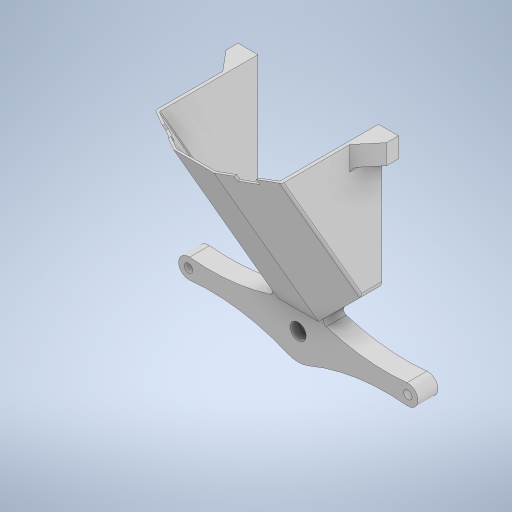
# Autodesk Inventor part: Brida_Rodamiento_Inferior
Saved by Autodesk Inventor 2024 (Build 280153000, 153)
## iProperties
Created: 2024-07-16
Part Number: Brida_Rodamiento_Inferior
Material: Genérico
Document SubType Name: Modeling
Designer: sergi
Density: 1 g/cm^3
Appearance: Valor por defecto
Author: sergi
Autodesk Inventor part; units mm, degrees
sketch "Boceto1" plane through (0, 0, 0) normal (0, 0, 1) x (1, 0, 0)
  circle A0 centre (0, 0) radius 8.25
  arc A1 (-36.764317, -25.949663) -> (36.764317, -25.949663) centre (0, 0) ccw
  arc A2 (-35.575624, -20.539596) -> (-36.764317, -25.949663) centre (-33.700624, -23.787191) ccw
  line L0 (-35.575624, -20.539596) -> (-15.909903, -9.185587)
  arc A3 (-11.227922, -9.946545) -> (-15.909903, -9.185587) centre (-14.034903, -12.433182) ccw
  arc A4 (-11.227922, -9.946545) -> (11.227922, -9.946545) centre (0, 0) ccw
  arc A5 (15.909903, -9.185587) -> (11.227922, -9.946545) centre (14.034903, -12.433182) ccw
  line L1 (15.909903, -9.185587) -> (35.575624, -20.539596)
  arc A6 (36.764317, -25.949663) -> (35.575624, -20.539596) centre (33.700624, -23.787191) ccw
  line L2 (98, -98) -> (98, 98)
  line L3 (98, 98) -> (-98, 98)
  line L4 (-98, 98) -> (-98, -98)
  line L5 (-98, -98) -> (98, -98)
  circle A7 centre (0, 0) radius 4
  line L6 (21.465456, -12.393087) -> (15.909903, -9.185587)
  arc A8 (15.909903, -9.185587) -> (11.227922, -9.946545) centre (14.034903, -12.433182) ccw
  arc A9 (-11.227922, -9.946545) -> (11.227922, -9.946545) centre (0, 0) ccw
  arc A10 (-11.227922, -9.946545) -> (-15.909903, -9.185587) centre (-14.034903, -12.433182) ccw
  line L7 (-15.909903, -9.185587) -> (-21.465456, -12.393087)
  line L8 (0, 0) -> (-55, 0) construction
  line L9 (0, 0) -> (55, 0) construction
  circle A11 centre (-55, 0) radius 2.1
  circle A12 centre (0, 0) radius 4
  circle A13 centre (-55, 0) radius 5
  circle A14 centre (0, 0) radius 13.4
  circle A15 centre (44.177818, -104.440798) radius 100
  circle A16 centre (-44.177818, -104.440798) radius 100
  arc A17 (0, 14.728367) -> (-5.220307, 12.341329) centre (-44.177818, 104.440798) ccw
  arc A18 (5.220307, 12.341329) -> (0, 14.728367) centre (44.177818, 104.440798) ccw
  line L10 (0, 0) -> (55, 0) construction
  circle A19 centre (55, 0) radius 5
  circle A20 centre (55, 0) radius 2.1
  line L11 (21.465456, -12.393087) -> (21.465456, 21.465456)
  line L12 (-21.465456, 21.465456) -> (-21.465456, -12.393087)
  line L13 (21.465456, 21.465456) -> (-21.465456, 21.465456)
  line L14 (-5.220307, 12.341329) -> (5.220307, 12.341329)
  line L15 (-11.631275, 9.885405) -> (11.631275, 9.885405)
  point P0 (0, 0)
  point P1 (21.81811, -12.596691)
  point P2 (-21.81811, -12.596691)
  point P3 (-11.631275, -9.46777)
  point P4 (-6.195652, 13.66067)
  point P5 (-54.484658, 4.973371)
  point P6 (-54.484658, -4.973371)
  point P7 (-14.969491, -8.801509)
  point P8 (14.969491, -8.801509)
  point P9 (6.195652, 13.66067)
  point P10 (27.999715, -35.228056)
  point P11 (-27.999715, -35.228056)
  point P12 (-11.125454, -10.061027)
  point P13 (11.125454, -10.061027)
  point P14 (11.227922, -9.946545)
  point P15 (11.227922, -9.946545)
  point P16 (54.484658, -4.973371)
  point P17 (54.484658, 4.973371)
  point P18 (25.599802, 0)
  point P19 (43.945653, 0)
  point P20 (-43.945653, 0)
  point P21 (-25.599802, 0)
  point P22 (-5.220307, -12.341329)
  point P23 (5.220307, -12.341329)
  point P24 (0, 192.73038)
  point P25 (0, 194.15323)
  point P26 (0, -194.15323)
  point P27 (0, -14.728367)
  point P28 (0.528736, -14.990678)
  point P29 (-0.528736, -14.990678)
  dimension "d3" = 180
  dimension "d4" = 4.2
  dimension "d16" = 10
  dimension "d18" = 55
  dimension "d19" = 26.8
  dimension "empalme" = 200
  dimension "d22" = 200
  dimension "d23" = 200
  dimension "d24" = 200
  dimension "d27" = 55
  dimension "d28" = 10
  dimension "d29" = 4.2
  constraints: 10 centre point, 10 end point, 8 point on circle, 8 tangent, 6 coincident, 3 horizontal, 1 collinear, 1 concentric, 1 point on line
  measures "d3" angle of L8 L9
  measures "d4" diameter of A11
  measures "d16" diameter of A13
  measures "d18" distance of L8.start L8.end
  measures "d19" diameter of A14
  measures "empalme" diameter of A15
  measures "d22" diameter of A16
  measures "d23" diameter of A17
  measures "d24" diameter of A18
  measures "d27" distance of L10.start L10.end
  measures "d28" diameter of A19
  measures "d29" diameter of A20
extrude "Extrusión1" add sketch "Boceto1" along normal blind 10 contours A0 | A15 L11 A18 A19 | A16 A3 A4 | A4 A3 A16 L12 A17 L15 A14 | A16 A13 A17 L12 | A15 A14 L15 A18 L11 A5 A4 | A4 A5 A15 | A14 L15 | A13 | A19
sketch "Boceto2" plane through (0, 0, 0) normal (0, 0, -1) x (-1, 0, 0)
  circle A0 centre (0, 0) radius 8.25 projected
  point P0 (0, 0)
extrude "Extrusión2" cut sketch "Boceto2" against normal blind 5
sketch "Boceto3" plane through (0, 0, 5) normal (0, 0, -1) x (-1, 0, 0)
  circle A0 centre (0, 0) radius 5.25 projected
  point P0 (0, 0)
extrude "Extrusión3" cut sketch "Boceto3" against normal blind 0.5
ref_plane "Plano de trabajo1" through (0, 0, 0) normal (0, 0, 1) x (1, 0, 0)
sketch "Boceto4" plane through (0, 0, 0) normal (0, 0, 1) x (1, 0, 0)
  line L0 (-31.810181, 100) -> (-31.810181, 32.452822)
  arc A0 (-31.810181, 32.452822) -> (-30.755766, 29.907238) centre (-28.210181, 32.452822) ccw
  line L1 (-30.755766, 29.907238) -> (-10.733933, 9.885405)
  line L2 (10.733933, 9.885405) -> (10.733933, 100)
  line L3 (30.755766, 29.907238) -> (30.755766, 100)
  line L4 (30.755766, 29.907238) -> (10.733933, 9.885405)
  line L5 (30.755766, 29.907238) -> (30.755766, 100)
  line L6 (-30.210181, 32.452822) -> (-30.210181, 100)
  arc A1 (-30.210181, 32.452822) -> (-29.624395, 31.038609) centre (-28.210181, 32.452822) ccw
  line L7 (-9.875898, 11.290112) -> (-29.624395, 31.038609)
  line L8 (9.875898, 11.290112) -> (-9.875898, 11.290112)
  line L9 (11.631275, 9.885405) -> (-11.631275, 9.885405)
  line L10 (29.624395, 31.038609) -> (9.875898, 11.290112)
  arc A2 (29.624395, 31.038609) -> (30.210181, 32.452822) centre (28.210181, 32.452822) ccw
  line L11 (30.210181, 100) -> (30.210181, 32.452822)
  line L12 (100, 100) -> (-100, 100)
  line L13 (31.810181, 32.452822) -> (31.810181, 100)
  arc A3 (30.755766, 29.907238) -> (31.810181, 32.452822) centre (28.210181, 32.452822) ccw
  line L14 (11.631275, 9.885405) -> (11.631275, 10.782746)
  line L15 (-11.631275, 9.885405) -> (-11.631275, 10.782746)
  point P0 (0, 0)
  point P1 (10.733933, 12.148146)
  constraints: 4 end point, 2 point on line, 1 parallel, 1 vertical
extrude "Extrusión4" add sketch "Boceto4" along normal up to surface (10 mm away) contours L12 L6 A1 L7 L8 L10 L2 L9 L1 A0 L0 | L1 L9 L15 | L10 A2 L11 L12 L3 L4 L2 | L4 L14 L9 | L12 L13 A3 L3
fillet "Empalme2" radius 2 4 edges at (-11.6313, 9.8854, 5) (-11.6313, 10.7827, 5) (11.6313, 9.8854, 5) (11.6313, 10.7827, 5)
sketch "Boceto5" plane through (0, 0, 10) normal (0, 0, 1) x (1, 0, 0)
  line L0 (-10.13864, 9.290112) -> (-30.755766, 29.907238)
  arc A0 (-31.810181, 32.452822) -> (-30.755766, 29.907238) centre (-28.210181, 32.452822) ccw
  arc A1 (-30.210181, 32.452822) -> (-29.624395, 31.038609) centre (-28.210181, 32.452822) ccw
  line L1 (-29.624395, 31.038609) -> (-9.875898, 11.290112)
  line L2 (-9.875898, 11.290112) -> (9.875898, 11.290112)
  line L3 (9.875898, 11.290112) -> (29.624395, 31.038609)
  line L4 (30.755766, 29.907238) -> (10.13864, 9.290112)
  arc A2 (30.755766, 29.907238) -> (31.810181, 32.452822) centre (28.210181, 32.452822) ccw
  line L5 (-103, 100) -> (100, 100)
  arc A3 (-54.484658, 4.973371) -> (-11.631275, 9.885405) centre (-44.177818, 104.440798) ccw
  arc A4 (-54.484658, 4.973371) -> (-11.631275, 9.885405) centre (-44.177818, 104.440798) ccw
  arc A5 (13.415067, 9.290112) -> (54.484658, 4.973371) centre (44.177818, 104.440798) ccw
  line L6 (11.631275, 10.782746) -> (11.631275, 9.885405)
  line L7 (-11.631275, 9.885405) -> (-11.631275, 10.782746)
  arc A6 (-54.484658, 4.973371) -> (-14.064455, 9.082603) centre (-44.177818, 104.440798) ccw
  arc A7 (-54.484658, 4.973371) -> (-54.484658, -4.973371) centre (-55, 0) ccw
  arc A8 (-5.220307, -12.341329) -> (-54.484658, -4.973371) centre (-44.177818, -104.440798) ccw
  arc A9 (-5.220307, -12.341329) -> (5.220307, -12.341329) centre (0, 0) ccw
  arc A10 (54.484658, -4.973371) -> (5.220307, -12.341329) centre (44.177818, -104.440798) ccw
  arc A11 (54.484658, -4.973371) -> (54.484658, 4.973371) centre (55, 0) ccw
  arc A12 (14.064455, 9.082603) -> (54.484658, 4.973371) centre (44.177818, 104.440798) ccw
  circle A13 centre (0, 0) radius 4
  line L8 (-14.064455, 9.082603) -> (-14.015792, 9.098659)
  line L9 (0, 11.290112) -> (0, 9.290112)
  line L10 (0, 9.290112) -> (-13.415067, 9.290112)
  line L11 (0, 9.290112) -> (13.415067, 9.290112)
  line L12 (30.755766, 29.907238) -> (13.252509, 12.403981)
  arc A14 (30.755766, 29.907238) -> (31.810181, 32.452822) centre (28.210181, 32.452822) ccw
  line L13 (31.810181, 100) -> (31.810181, 32.452822)
  line L14 (30.210181, 100) -> (31.810181, 100)
  line L15 (30.210181, 32.452822) -> (30.210181, 100)
  arc A15 (29.624395, 31.038609) -> (30.210181, 32.452822) centre (28.210181, 32.452822) ccw
  line L16 (9.875898, 11.290112) -> (29.624395, 31.038609)
  line L17 (-9.875898, 11.290112) -> (9.875898, 11.290112)
  line L18 (-29.624395, 31.038609) -> (-9.875898, 11.290112)
  arc A16 (-30.210181, 32.452822) -> (-29.624395, 31.038609) centre (-28.210181, 32.452822) ccw
  line L19 (-30.210181, 100) -> (-30.210181, 32.452822)
  line L20 (-31.810181, 100) -> (-30.210181, 100)
  line L21 (-31.810181, 32.452822) -> (-31.810181, 100)
  arc A17 (-31.810181, 32.452822) -> (-30.755766, 29.907238) centre (-28.210181, 32.452822) ccw
  line L22 (-13.252509, 12.403981) -> (-30.755766, 29.907238)
  arc A18 (-14.064455, 9.082603) -> (-13.252509, 12.403981) centre (-14.666723, 10.989767) ccw
  arc A19 (13.252509, 12.403981) -> (14.064455, 9.082603) centre (14.666723, 10.989767) ccw
  point P0 (0, 0)
  point P1 (-31.810181, 100)
  point P2 (-30.210181, 100)
  point P3 (30.210181, 100)
  point P4 (31.810181, 100)
  point P5 (-31.810181, 32.452822)
  dimension "d59" = 2
  constraints: 12 end point, 4 point on circle, 2 point on line, 1 centre point, 1 horizontal, 1 perpendicular
  measures "d59" distance of L9.start L9.end
ref_plane "Plano de trabajo2" through (0, 32.452822, 0) normal (-1, 0, 0) x (0, 0, 1)
sketch "Boceto6" plane through (0, 32.452822, 0) normal (-1, 0, 0) x (0, 0, 1)
  line L0 (10, -23.16271) -> (81, 99.812897)
  point P0 (10, 67.547178)
  constraints: 2 end point
sweep "Barrido1" add profiles "Boceto5" path "Boceto6" contours L0 A0 L21 L5 L19 A1 L1 L2 L9 L10 | L9 L2 L3 A15 L15 L5 L13 A2 L4 L11
ref_plane "Plano de trabajo3" through (-31.810181, 100, 0) normal (0, 1, 0) x (1, 0, 0)
split "Dividir1" plane through (-31.810181, 100, 0) removes the side toward (0, 1, 0)
sketch "Boceto7" plane through (-31.810181, 32.452822, 0) normal (-1, 0, 0) x (0, 0, 1)
  line L0 (0, 67.547178) -> (48.998381, 67.547178)
  line L1 (0, 67.547178) -> (0, 0)
  line L2 (0, 0) -> (10, 0)
  line L3 (0, 67.547178) -> (16, 67.547178)
  line L4 (16, 67.547178) -> (16, 57.547178)
  line L5 (16, 57.547178) -> (0, 57.547178)
  line L6 (0, 57.547178) -> (0, 67.547178)
  line L7 (10, 0) -> (48.998381, 67.547178)
  point P0 (0, -32.452822)
  point P1 (0, 57.547178)
  point P2 (16, 67.547178)
  point P3 (16, 67.547178)
  dimension "d41" = 10
  dimension "d56" = 16
  constraints: 8 end point, 2 parallel, 1 horizontal, 1 perpendicular
  measures "d41" distance of L3.end L4.end
  measures "d56" distance of L4.end L5.end
extrude "Extrusión5" add sketch "Boceto7" along normal blind 8.4 contours L0 L4 L5 L1
chamfer "Chaflán2" distance 10 distance2 8.4 1 edges at (-40.2102, 95, 16) measured on face at (-40.2102, 96.6667, 10.6667)
sketch "Boceto8" plane through (0, 0, 0) normal (0, 0, -1) x (-1, 0, 0)
  line L0 (30.210181, 100) -> (-31.810181, 100)
  line L1 (30.210181, 32.452822) -> (30.210181, 100)
  line L2 (40.210181, 100) -> (40.210181, 90)
  line L3 (-98, 100) -> (100, 100)
  line L4 (31.810181, 90) -> (40.210181, 90)
  line L5 (31.810181, 90) -> (31.810181, 32.452822)
  circle A0 centre (35, 95) radius 2.1
  point P0 (0, 0)
  point P1 (25.210181, 95)
  point P2 (31.810181, 100)
  dimension "d47" = 5
  dimension "d55" = 5
  dimension "d62" = 4.2
  constraints: 1 centre point
  measures "d47" distance from line of L0 point (25.21, 95)
  measures "d55" distance from line of L1 point (25.21, 95)
  measures "d62" diameter of A0
hole "Agujero1" at (-35, 95, 0) direction (0, 0, 1) diameter 4.2 depth 4
ref_plane "Plano de trabajo4" through (0, 32.452822, 0) normal (-1, 0, 0) x (0, 0, 1)
mirror "Simetría1" about plane through (0, 32.452822, 0) normal (-1, 0, 0) of "Extrusión5", "Chaflán2", "Agujero1"
fillet "Empalme1" radius 2 4 edges at (-31.8102, 90, 16) (-31.8102, 90, 8) (31.8102, 90, 16) (31.8102, 90, 8)
sketch "Boceto9" plane through (-10.13864, 100, 62.371378) normal (0, 1, 0) x (1, 0, 0)
  line L0 (-89.86136, 115.371378) -> (-92.86136, 115.371378)
  line L1 (-92.86136, 115.371378) -> (-92.86136, 90.371378)
  line L2 (-92.86136, 90.371378) -> (-89.86136, 90.371378)
  line L3 (-89.86136, 90.371378) -> (-89.86136, 65.371378)
  line L4 (-89.86136, 65.371378) -> (-92.86136, 65.371378)
  line L5 (-92.86136, 65.371378) -> (-92.86136, 40.371378)
  line L6 (-92.86136, 40.371378) -> (-89.86136, 40.371378)
  line L7 (-89.86136, 40.371378) -> (-89.86136, 15.371378)
  line L8 (-89.86136, 15.371378) -> (-92.86136, 15.371378)
  line L9 (-92.86136, 15.371378) -> (-92.86136, -9.628622)
  line L10 (-92.86136, -9.628622) -> (-89.86136, -9.628622)
  line L11 (-89.86136, -9.628622) -> (-89.86136, -34.628622)
  line L12 (-89.86136, -34.628622) -> (-92.86136, -34.628622)
  line L13 (-92.86136, -34.628622) -> (-92.86136, -59.628622)
  line L14 (-92.86136, -59.628622) -> (-89.86136, -59.628622)
  line L15 (-89.86136, -59.628622) -> (-89.86136, -84.628622)
  line L16 (-89.86136, -84.628622) -> (-14.86136, -84.628622)
  line L17 (113.13864, -84.628622) -> (113.13864, -59.628622)
  line L18 (113.13864, -59.628622) -> (110.13864, -59.628622)
  line L19 (110.13864, -59.628622) -> (110.13864, -34.628622)
  line L20 (110.13864, -34.628622) -> (113.13864, -34.628622)
  line L21 (113.13864, -34.628622) -> (113.13864, -9.628622)
  line L22 (113.13864, -9.628622) -> (110.13864, -9.628622)
  line L23 (110.13864, -9.628622) -> (110.13864, 15.371378)
  line L24 (110.13864, 15.371378) -> (113.13864, 15.371378)
  line L25 (113.13864, 15.371378) -> (113.13864, 40.371378)
  line L26 (113.13864, 40.371378) -> (110.13864, 40.371378)
  line L27 (110.13864, 40.371378) -> (110.13864, 65.371378)
  line L28 (110.13864, 65.371378) -> (113.13864, 65.371378)
  line L29 (113.13864, 65.371378) -> (113.13864, 90.371378)
  line L30 (113.13864, 90.371378) -> (110.13864, 90.371378)
  line L31 (110.13864, 90.371378) -> (110.13864, 115.371378)
  line L32 (110.13864, 115.371378) -> (113.13864, 115.371378)
  line L33 (113.13864, 115.371378) -> (113.13864, 140.371378)
  line L34 (113.13864, 140.371378) -> (110.13864, 140.371378)
  line L35 (110.13864, 140.371378) -> (110.13864, 165.371378)
  line L36 (110.13864, 165.371378) -> (-92.86136, 165.371378)
  line L37 (-92.86136, 165.371378) -> (-92.86136, 140.371378)
  line L38 (-92.86136, 140.371378) -> (-89.86136, 140.371378)
  line L39 (-89.86136, 140.371378) -> (-89.86136, 115.371378)
  circle A0 centre (-39.86136, 150.371378) radius 1.75
  circle A1 centre (60.13864, 150.371378) radius 1.75
  circle A2 centre (60.13864, -72.628622) radius 1.5
  circle A3 centre (-39.86136, -72.628622) radius 1.5
  circle A4 centre (-39.86136, 50.371378) radius 1.5
  circle A5 centre (60.13864, 50.371378) radius 1.5
  line L40 (31.68168, 7.890728) -> (31.68168, -2.975298)
  line L41 (31.68168, -2.975298) -> (28.68168, -2.975298)
  line L42 (28.68168, -2.975298) -> (28.68168, 6.158677)
  line L43 (28.68168, 6.158677) -> (20.014539, 1.154701)
  line L44 (20.014539, 1.154701) -> (0.262742, 1.154701)
  line L45 (0.262742, 1.154701) -> (-8.4044, 6.158677)
  line L46 (-8.4044, 6.158677) -> (-8.4044, -2.975298)
  line L47 (-8.4044, -2.975298) -> (-11.4044, -2.975298)
  line L48 (-11.4044, -2.975298) -> (-11.4044, 7.890728)
  line L49 (-11.4044, 7.890728) -> (-19.485755, 12.5565)
  ellipse E0 centre (-18.071541, 13.372997) end of major axis (-16.071541, 13.372997) minor radius 1.154701 (-20.071541, 13.372997) -> (-19.485755, 12.5565) ccw
  line L50 (-20.071541, 13.372997) -> (-20.071541, 23.372997)
  line L51 (-20.071541, 23.372997) -> (40.348822, 23.372997)
  line L52 (40.348822, 23.372997) -> (40.348822, 13.372997)
  ellipse E1 centre (38.348822, 13.372997) end of major axis (40.348822, 13.372997) minor radius 1.154701 (39.763035, 12.5565) -> (40.348822, 13.372997) ccw
  line L53 (39.763035, 12.5565) -> (31.68168, 7.890728)
  line L54 (-6.4044, -4.975298) -> (-6.4044, 2.694575)
  line L55 (-6.4044, 2.694575) -> (-0.273157, -0.845299)
  line L56 (-0.273157, -0.845299) -> (20.550437, -0.845299)
  line L57 (20.550437, -0.845299) -> (26.68168, 2.694575)
  line L58 (26.68168, 2.694575) -> (26.68168, -4.975298)
  line L59 (26.68168, -4.975298) -> (33.68168, -4.975298)
  line L60 (33.68168, -4.975298) -> (33.68168, 6.736027)
  line L61 (33.68168, 6.736027) -> (40.763035, 10.82445)
  line L62 (42.348822, 13.372997) -> (42.348822, 25.372997)
  line L63 (42.348822, 25.372997) -> (-22.071541, 25.372997)
  line L64 (-22.071541, 25.372997) -> (-22.071541, 13.372997)
  line L65 (-20.485755, 10.82445) -> (-13.4044, 6.736027)
  line L66 (-13.4044, 6.736027) -> (-13.4044, -4.975298)
  line L67 (-13.4044, -4.975298) -> (-6.4044, -4.975298)
  line L68 (-13.4044, 6.736027) -> (-13.4044, 14)
  line L69 (-13.4044, 14) -> (-6.4044, 14)
  line L70 (-6.4044, 14) -> (-6.4044, 2.694575)
  line L71 (26.68168, -4.975298) -> (33.68168, -4.975298)
  line L72 (33.68168, -4.975298) -> (33.68168, 14)
  line L73 (33.68168, 14) -> (26.68168, 14)
  line L74 (26.68168, 14) -> (26.68168, -4.975298)
  line L75 (32.13864, -84.628622) -> (32.13864, -69.628622)
  line L76 (32.13864, -69.628622) -> (35.13864, -69.628622)
  line L77 (35.13864, -69.628622) -> (35.13864, -84.628622)
  line L78 (35.13864, -84.628622) -> (113.13864, -84.628622)
  line L79 (-14.86136, -84.628622) -> (-14.86136, -69.628622)
  line L80 (-14.86136, -69.628622) -> (-11.86136, -69.628622)
  line L81 (-11.86136, -69.628622) -> (-11.86136, -84.628622)
  line L82 (2.63864, -84.628622) -> (2.63864, -74.628622)
  line L83 (2.63864, -74.628622) -> (17.63864, -74.628622)
  line L84 (17.63864, -74.628622) -> (17.63864, -84.628622)
  line L85 (17.63864, -84.628622) -> (32.13864, -84.628622)
  line L86 (-11.86136, -84.628622) -> (2.63864, -84.628622)
  spline S0 degree 4 poles (40.763034, 10.824452) (41.072078, 11.002803) (41.359361, 11.219056) (41.919869, 11.784102) (42.256137, 12.512862) (42.348694, 12.942835) (42.348836, 13.372997) knots 0 0 0 0 0 0.45346504 0.45346504 1 1 1 1 1
  spline S1 degree 4 poles (-22.071556, 13.372997) (-22.071414, 12.942835) (-21.978856, 12.512862) (-21.642589, 11.784102) (-21.082081, 11.219056) (-20.794797, 11.002803) (-20.485753, 10.824452) knots 0 0 0 0 0 0.54653496 0.54653496 1 1 1 1 1
  point P0 (10.13864, 62.371378)
  point P1 (26.68168, 2.694575)
  point P2 (33.68168, 4.33303)
  point P3 (33.68168, 4.736027)
  point P4 (26.68168, 2.694575)
  point P5 (33.68168, 6.736027)
  dimension "d63" = 2
  constraints: 42 end point, 6 parallel, 3 perpendicular, 1 horizontal, 1 vertical, 19 other
  measures "d63" distance between parallel lines of L46 L54
extrude "Extrusión6" cut sketch "Boceto9" against normal blind 3 contours L53 L72 L60 L59 L58 L74 L43 L42 L41 L40 | L40 L41 L42 L43 L74 L73 L72 L53 | L70 L54 L67 L66 L68 L49 L48 L47 L46 L45 | L45 L46 L47 L48 L49 L68 L69 L70
equation "\"d22\" = empalme"
equation "\"d23\" = empalme"
equation "\"d24\" = empalme"
